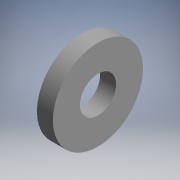
# Autodesk Inventor part: 25-2281_p2
Saved by Autodesk Inventor 2017.3 (Build 213256000, 256)
## iProperties
Part Number: 25-2281_p2
Material: Generic
Catalog Web Link: www.cadenas.de
Description: 25-2281, 65-2282, 40-2280, 40-2290_p2-Roller Wheels
Vendor: 8020
Document SubType Name: Modeling
Designer: partserver
Manufacturer: 8020
Mass: 0.46023 g
Surface Area: 5.23567 cm^2
Volume: 0.46023 cm^3
Density: 1 g/cm^3
Appearance: PSOLRGB-192-192-192
Category: PARTsolutions
Company: 8020
Title: 25-2281_p2
Author: Cadenas PARTsolutions
Comments: Roller Wheels
PSOL_IDENT_0: {$CADENAS_DATA\23d-libs\8020\metric\linear_motion\25_2281_p2.prj},196 {VTYP=3D},{NB=25-2281_p2},{LIN
PSOL_IDENT_1: A=25-2281_p2},{NN=25-2281, 65-2282, 40-2280, 40-2290_p2},{DATE=31.07.2020 09:21:29},{GEOMDATE=22.03.
PSOL_IDENT_2: 2012 00:00:00},{VERSION=},{LINEID=10},{WBVAR=BT,RI},{WBNUMERIC=}  {NB=25-2281_p2},{LINA=25-2281_p2},
PSOL_IDENT_3: {KT=DUMMY},{PN=25-2281},{NO=1},{MAT=Self-lubricating, fiberglass-reinforced black nylon.},{BT=2},{BT
PSOL_IDENT_4: 1= '2','Permanent Lubricated Bronze Bushing' },{MT=25 Series},{RI=25},{RI1= '25','25 Series','40','4
PSOL_IDENT_5: 0 Series' },{A=37.500},{B=28.000},{C=6.100},{D=12.000},{E=14.000},{F=4.750},{G=8.000},{H=5.500},{J=2
PSOL_IDENT_6: .80000000},{K=15.79880},{L=13.200},{M=8.65000000},{N=M6 x 1.0},{N1=6.3500},{P=1.600},{Q=9.200},{W=.0
PSOL_IDENT_7: 32},{G1=10.000},{K1=0.000},{NTP=3382},{WF=4.08400},{T=3.30000}
NB: 25-2281_p2
NN: 25-2281, 65-2282, 40-2280, 40-2290_p2
NT: Roller Wheels
NBSYN: $PN._p2
LINA: 25-2281_p2
CATALOG: 80/20
NO: 1
MAT: Self-lubricating, fiberglass-reinforced black nylon.
BT: Permanent Lubricated Bronze Bushing
MT: 25 Series
RI: 25 Series
A: 37.5
B: 28
D: 12
E: 14
F: 4.75
G: 8
H: 5.5
J: 2.8
K: 15.7988
L: 13.2
M: 8.65
N: M6 x 1.0
N1: 6.35
P: 1.6
Q: 9.2
K1: 0
NTP: 3382
WF: 4.084
T: 3.3
SUPPLIER: 8020
ARTICLENO: 25-2281_p2
BOMINFO: 25-2281_p2
CREATOR: CADENAS GmbH
Autodesk Inventor part; units mm, degrees
ref_plane "YZ Plane" through (0, 0, 0) normal (1, 0, 0) x (0, 1, 0)
ref_plane "XZ Plane" through (0, 0, 0) normal (0, 1, 0) x (-1, 0, 0)
ref_plane "XY Plane" through (0, 0, 0) normal (0, 0, 1) x (1, 0, 0)
sketch "Sketch_1" plane through (0, 0, 0) normal (0, 0, 1) x (1, 0, 0)
  line L0 (1.4, 0) -> (-1.4, 0)
  line L1 (-1.4, 3.175) -> (1.4, 3.175)
  line L2 (1.4, 3.175) -> (1.4, 7.8994)
  line L3 (1.4, 7.8994) -> (-1.4, 7.8994)
  line L4 (-1.4, 7.8994) -> (-1.4, 3.175)
  constraints: 10 end point
revolve "Revolution1" add sketch "Sketch_1" angle 360 about axis through (1.4, 0, 0) along (1, 0, 0)
ref_plane "P2_XY" through (1.4, 0, 0) normal (1, 0, 0) x (0, 0, -1)
ref_plane "P2_YZ" through (1.4, 0, 0) normal (0, 0, -1) x (0, 1, 0)
ref_plane "P2_ZX" through (1.4, 0, 0) normal (0, 1, 0) x (1, 0, 0)
body "Solid1"
